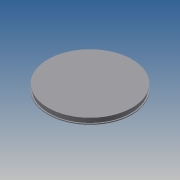
# Autodesk Inventor part: distal idler pulley special
Saved by Autodesk Inventor 2013 (Build 170138000, 138)
## iProperties
Created: 2017-03-06
Part Number: distal idler pulley special
Material: Generic
Document SubType Name: Modeling
Designer: employee
Density: 1 g/cm^3
Author: employee
Autodesk Inventor part; units mm, degrees
ref_plane "YZ Plane" through (0, 0, 0) normal (1, 0, 0) x (0, 1, 0)
ref_plane "XZ Plane" through (0, 0, 0) normal (0, 1, 0) x (-1, 0, 0)
ref_plane "XY Plane" through (0, 0, 0) normal (0, 0, 1) x (1, 0, 0)
sketch "Sketch1" plane through (0, 0, 0) normal (0, 0, 1) x (1, 0, 0)
  circle A0 centre (0, 0) radius 33
  dimension "d0" = 66
  constraints: 1 centre point, 1 coincident
  measures "d0" diameter of A0
extrude "Extrusion1" add sketch "Sketch1" along normal blind 1.5
sketch "Sketch2" plane through (0, 0, 1.5) normal (0, 0, 1) x (1, 0, 0)
  circle A0 centre (0, 0) radius 33 projected
  circle A1 centre (0, 0) radius 31
  dimension "d15" = 2
  constraints: 1 centre point, 1 coincident
  measures "d15" radial gap between concentric circles of A0 A1
extrude "Extrusion2" add sketch "Sketch2" along normal blind 7 contours A1
sketch "Sketch3" plane through (0, 0, 8.5) normal (0, 0, 1) x (1, 0, 0)
  circle A0 centre (0, 0) radius 33 projected
  circle A1 centre (0, 0) radius 31 projected
  circle A2 centre (0, 0) radius 77
  dimension "d16" = 154
  constraints: 1 centre point, 1 coincident
  measures "d16" diameter of A2
extrude "Extrusion3" add sketch "Sketch3" along normal blind 1.5 contours A0 | A1 | A2
sketch "Sketch5" plane through (0, 0, 10) normal (0, 0, 1) x (1, 0, 0)
  circle A0 centre (0, 0) radius 77 projected
  circle A1 centre (0, 0) radius 75
  dimension "d18" = 150
  constraints: 1 centre point, 1 coincident
  measures "d18" diameter of A1
extrude "Extrusion5" add sketch "Sketch5" along normal blind 7 contours A1
sketch "Sketch6" plane through (0, 0, 17) normal (0, 0, 1) x (1, 0, 0)
  circle A0 centre (0, 0) radius 77 projected
extrude "Extrusion6" add sketch "Sketch6" along normal blind 1.5
sketch "Sketch4" plane through (0, 0, 0) normal (0, 0, -1) x (-1, 0, 0)
  circle A0 centre (0, 0) radius 33 projected
  line L0 (30.541, 12.5) -> (0, 12.5)
  arc A1 (0, 12.5) -> (0, -12.5) centre (0, 0) ccw
  line L1 (0, -12.5) -> (30.541, -12.5)
  dimension "d10" = 12.5
  constraints: 4 end point, 4 point on circle, 2 horizontal, 2 tangent, 1 centre point, 1 concentric
  measures "d10" radius of A1
body "Solid1"
